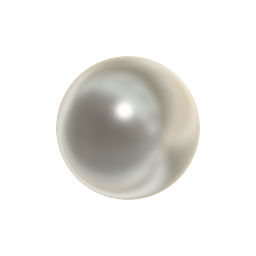
Baby REPO (Autodesk Fusion 360 archive; units mm, degrees)
design "Ojo repo"
Autodesk Fusion 360 part; units mm, degrees
(part 1 of 2)
sphere "EsferaPrimitiva1" add diameter 13 placed x (0, 1, 0) y (0, 0, 1) z (1, 0, 0) at (0, 0, 0)
sketch "Boceto2" plane through (0, 0, 0) normal (0, 1, 0) x (1, 0, 0)
  circle A0 centre (0, 0) radius 20
  dimension "d2" = 40
  constraint coincident A0.centre origin
  measures "d2" diameter of A0
sketch "Boceto1" plane through (0, 0, 0) normal (0, 1, 0) x (1, 0, 0)
  circle A0 centre (0, 0) radius 10
  line L0 (0, 0) -> (0, -13.2142)
  dimension "d1" = 20
  constraint coincident A0.centre L0.start
  constraint vertical L0
  measures "d1" diameter of A0

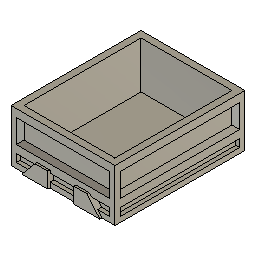
design "Carro"
Autodesk Fusion 360 part; units mm, degrees
sketch "Sketch1" plane through (0, 0, 0) normal (0, 0, 1) x (1, 0, 0)
  line L0 (20, -25) -> (-20, -25)
  line L1 (-20, -25) -> (-20, 25)
  line L2 (-20, 25) -> (20, 25)
  line L3 (20, 25) -> (20, -25)
  line L4 (20, -25) -> (-20, 25) construction
  line L5 (-20, -25) -> (20, 25) construction
  dimension "d1" = 40
  dimension "d2" = 50
  constraint horizontal L0
  constraint perpendicular L0 L1
  constraint parallel L0 L2
  constraint parallel L1 L3
  constraint coincident L4 origin
  constraint coincident L5 origin
  measures "d1" distance of L1.end L2.end
  measures "d2" distance of L0.end L1.end
extrude "Extrude1" add sketch "Sketch1" along normal blind 20
sketch "Sketch2" plane through (0, 25, 0) normal (0, 1, 0) x (-1, 0, 0)
  line L0 (-20, 0) -> (20, 0)
  line L1 (20, 0) -> (20, 20)
  line L2 (20, 20) -> (-20, 20)
  line L3 (-20, 20) -> (-20, 0)
  line L4 (0, 9) -> (0, 20) construction
  line L5 (0, 9) -> (0, 8) construction
  line L6 (0, 8) -> (18, 8)
  line L7 (18, 8) -> (18, 17)
  line L8 (18, 17) -> (-18, 17)
  line L9 (-18, 17) -> (-18, 8)
  line L10 (-18, 8) -> (0, 8)
  line L11 (-18, 8) -> (-18, 2) construction
  line L12 (-18, 2) -> (18, 2) construction
  line L13 (18, 2) -> (18, 8) construction
  line L14 (-18, 2) -> (18, 2)
  line L15 (18, 2) -> (18, 5)
  line L16 (18, 5) -> (-18, 5)
  line L17 (-18, 5) -> (-18, 2)
  line L18 (20, 0) -> (20, 20)
  dimension "d5" = 3
  dimension "d8" = 2
  dimension "d9" = 6
  dimension "d13" = 2
  dimension "d43" = 2
  constraint midpoint L2 L4.end
  constraint perpendicular L0 L4
  constraint coincident L4 L5.end
  constraint perpendicular L5 L6
  constraint perpendicular L6 L7
  constraint perpendicular L4 L8
  constraint perpendicular L6 L9
  constraint perpendicular L5 L10
  constraint perpendicular L10 L11
  constraint perpendicular L11 L12
  constraint perpendicular L12 L13
  constraint horizontal L14
  constraint vertical L15
  constraint horizontal L16
  constraint vertical L17
  constraint midpoint L13 L15.end
  measures "d5" distance of L2 L8
  measures "d8" distance of L3 L9
  measures "d9" distance of L6.end L12.end
  measures "d13" distance of L0 L12
  measures "d43" distance of L7 L18
sketch "Sketch3" plane through (-20, 0, 0) normal (-1, 0, 0) x (0, -1, 0)
  line L0 (-25, 0) -> (25, 0)
  line L1 (25, 0) -> (25, 20)
  line L2 (25, 20) -> (-25, 20)
  line L3 (-25, 20) -> (-25, 0)
  line L4 (-23, 17) -> (23, 17)
  line L5 (23, 17) -> (23, 8)
  line L6 (23, 8) -> (-23, 8)
  line L7 (-23, 8) -> (-23, 17)
  line L8 (-23, 5) -> (23, 5)
  line L9 (23, 5) -> (23, 2)
  line L10 (23, 2) -> (-23, 2)
  line L11 (-23, 2) -> (-23, 5)
  dimension "d14" = 3
  dimension "d15" = 2
  dimension "d16" = 2
  dimension "d18" = 2
  dimension "d19" = 2
  dimension "d20" = 6
  dimension "d21" = 3
  dimension "d22" = 2
  constraint horizontal L4
  constraint vertical L5
  constraint horizontal L6
  constraint vertical L7
  constraint horizontal L8
  constraint vertical L9
  constraint horizontal L10
  constraint vertical L11
  measures "d14" distance of L2 L4
  measures "d15" distance of L1 L5
  measures "d16" distance of L3 L7
  measures "d18" distance of L1 L9
  measures "d19" distance of L3 L11
  measures "d20" distance of L6 L10
  measures "d21" distance of L8 L10
  measures "d22" distance of L0 L10
sketch "Sketch4" plane through (20, 0, 0) normal (1, 0, 0) x (0, 1, 0)
  line L0 (-25, 0) -> (25, 0)
  line L1 (25, 0) -> (25, 20)
  line L2 (25, 20) -> (-25, 20)
  line L3 (-25, 20) -> (-25, 0)
  line L4 (-23, 8) -> (23, 8)
  line L5 (23, 8) -> (23, 17)
  line L6 (-23, 17) -> (-23, 8)
  line L7 (23, 17) -> (-23, 17)
  line L8 (-23, 2) -> (23, 2)
  line L9 (23, 2) -> (23, 5)
  line L10 (-23, 5) -> (-23, 2)
  line L11 (23, 5) -> (-23, 5)
sketch "Sketch5" plane through (0, -25, 0) normal (0, -1, 0) x (1, 0, 0)
  line L0 (-20, 0) -> (20, 0)
  line L1 (20, 0) -> (20, 20)
  line L2 (20, 20) -> (-20, 20)
  line L3 (-20, 20) -> (-20, 0)
  line L4 (-18, 8) -> (-18, 17)
  line L5 (-18, 17) -> (18, 17)
  line L6 (18, 17) -> (18, 8)
  line L7 (0, 8) -> (-18, 8)
  line L8 (18, 8) -> (0, 8)
  line L9 (18, 2) -> (-18, 2)
  line L10 (-18, 2) -> (-18, 5)
  line L11 (18, 5) -> (18, 2)
  line L12 (-18, 5) -> (18, 5)
extrude "Extrude2" cut sketch "Sketch2" against normal blind 1.5 contours L6 L7 L8 L9 L10 | L14 L15 L16 L17
extrude "Extrude3" cut sketch "Sketch3" against normal blind 1.5 contours L4 L5 L6 L7 | L8 L9 L10 L11
extrude "Extrude4" cut sketch "Sketch5" against normal blind 1.5 contours L4 L5 L6 L7 L8 | L9 L10 L11 L12
extrude "Extrude5" cut sketch "Sketch4" against normal blind 1.5 contours L4 L5 L6 L7 | L8 L9 L10 L11
chamfer "Chamfer1" distance 1.5 angle 45 5 edges at (18, 23.5, 12.5) (0, 23.5, 17) (-18, 23.5, 12.5) (0, 23.5, 8) (18.5, 0, 8) 3 faces at (18.5, -7.6667, 14) (-6, -23.5, 14) (-18.5, 7.6667, 14)
sketch "Sketch6" plane through (0, 0, 20) normal (0, 0, 1) x (-1, 0, 0)
  line L0 (-20, -25) -> (20, -25)
  line L1 (20, -25) -> (20, 25)
  line L2 (20, 25) -> (-20, 25)
  line L3 (-20, 25) -> (-20, -25)
  line L4 (-17.5, 22.5) -> (17.5, 22.5)
  line L5 (17.5, 22.5) -> (17.5, -22.5)
  line L6 (17.5, -22.5) -> (-17.5, -22.5)
  line L7 (-17.5, -22.5) -> (-17.5, 22.5)
  line L8 (-17.5, 22.5) -> (17.5, -22.5) construction
  line L9 (17.5, 22.5) -> (-17.5, -22.5) construction
  dimension "d29" = 2.5
  dimension "d30" = 2.5
  constraint horizontal L4
  constraint perpendicular L4 L5
  constraint parallel L4 L6
  constraint parallel L5 L7
  constraint coincident L8 origin
  constraint coincident L9 origin
  measures "d29" distance of L3 L7
  measures "d30" distance of L0 L6
extrude "Extrude6" cut sketch "Sketch6" against normal blind 18 contours L4 L5 L6 L7
sketch "Sketch7" plane through (0, -25, 0) normal (0, -1, 0) x (1, 0, 0)
  line L0 (18, 2) -> (-18, 2)
  line L1 (-18, 5) -> (18, 5)
  line L2 (18, 5) -> (18, 2)
  line L3 (-20, 0) -> (20, 0)
  line L4 (20, 0) -> (20, 20)
  line L5 (20, 20) -> (-20, 20)
  line L6 (-20, 20) -> (-20, 0)
  line L7 (0, 0) -> (0, 20)
  line L8 (0, 0) -> (-5, 0) construction
  line L9 (-5, 0) -> (-5, 6)
  line L10 (-5, 6) -> (-10, 6)
  line L11 (-10, 6) -> (-15, 0)
  line L12 (-5, 0) -> (-15, 0)
  line L13 (10, 6) -> (15, 0)
  line L14 (5, 0) -> (15, 0)
  line L15 (5, 6) -> (10, 6)
  line L16 (5, 0) -> (5, 6)
  line L17 (-18, 17) -> (18, 17)
  line L18 (18, 17) -> (18, 8)
  line L19 (18, 8) -> (-18, 8)
  line L20 (-18, 8) -> (-18, 17)
  line L21 (-18, 2) -> (-18, 5)
  dimension "d33" = 6
  dimension "d34" = 5
  dimension "d35" = 10
  dimension "d36" = 5
  constraint coincident L7.start L8.start
  constraint midpoint L5 L7.end
  constraint coincident L3 L8.end
  constraint perpendicular L1 L9
  constraint perpendicular L9 L10
  constraint coincident L3 L11.end
  constraint symmetric L7 L8.end L14.start
  constraint symmetric L7 L9.end L15.start
  constraint symmetric L7 L10.end L13.start
  constraint symmetric L7 L11.end L13.end
  measures "d33" distance of L8.end L9.end
  measures "d34" distance of L9.end L10.end
  measures "d35" distance of L8.end L11.end
  measures "d36" distance of L7.start L8.end
extrude "Extrude7" add sketch "Sketch7" along normal blind 0.8 and the other way blind 2 contours L0 L3 L13 L14 L16 | L0 L1 L13 L16 | L1 L13 L15 L16 | L0 L3 L9 L11 L12 | L0 L1 L9 L11 | L1 L9 L10 L11
mirror "Mirror1" about plane through (0, 0, 0) normal (0, 1, 0) of "Extrude7"
equation "a = -1.5 mm"
equation "d25 = a"
equation "d27 = a"

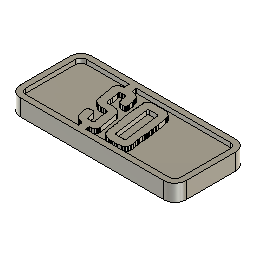
design "Placa"
Autodesk Fusion 360 part; units mm, degrees
sketch "Sketch1" plane through (0, 0, 0) normal (0, 0, 1) x (1, 0, 0)
  line L0 (15, -6.5) -> (-15, -6.5)
  line L1 (-15, -6.5) -> (-15, 6.5)
  line L2 (-15, 6.5) -> (15, 6.5)
  line L3 (15, 6.5) -> (15, -6.5)
  line L4 (15, -6.5) -> (-15, 6.5) construction
  line L5 (-15, -6.5) -> (15, 6.5) construction
  dimension "d1" = 30
  dimension "d2" = 13
  constraint horizontal L0
  constraint perpendicular L0 L1
  constraint parallel L0 L2
  constraint parallel L1 L3
  constraint coincident L4 origin
  constraint coincident L5 origin
  measures "d1" distance of L1.end L2.end
  measures "d2" distance of L0 L2
extrude "Extrude1" add sketch "Sketch1" along normal blind 3
fillet "Fillet1" radius 2 4 edges at (15, 6.5, 1.5) (15, -6.5, 1.5) (-15, 6.5, 1.5) (-15, -6.5, 1.5)
sketch "Sketch2" plane through (0, 0, 3) normal (0, 0, 1) x (-1, 0, 0)
  arc A0 (15, 4.5) -> (13, 6.5) centre (13, 4.5) ccw
  line L0 (13, 6.5) -> (-13, 6.5)
  arc A1 (-13, 6.5) -> (-15, 4.5) centre (-13, 4.5) ccw
  line L1 (-15, 4.5) -> (-15, -4.5)
  arc A2 (-15, -4.5) -> (-13, -6.5) centre (-13, -4.5) ccw
  line L2 (-13, -6.5) -> (13, -6.5)
  arc A3 (13, -6.5) -> (15, -4.5) centre (13, -4.5) ccw
  line L3 (15, -4.5) -> (15, 4.5)
  line L4 (14, -4.5) -> (14, 4.5)
  arc A4 (14, 4.5) -> (13, 5.5) centre (13, 4.5) ccw
  line L5 (13, 5.5) -> (-13, 5.5)
  arc A5 (-13, 5.5) -> (-14, 4.5) centre (-13, 4.5) ccw
  line L6 (-14, 4.5) -> (-14, -4.5)
  arc A6 (-14, -4.5) -> (-13, -5.5) centre (-13, -4.5) ccw
  line L7 (-13, -5.5) -> (13, -5.5)
  arc A7 (13, -5.5) -> (14, -4.5) centre (13, -4.5) ccw
  dimension "d10" = -1
extrude "Extrude2" cut sketch "Sketch2" against normal blind 0.8 contours L4 A4 L5 A5 L6 A6 L7 A7
sketch "Sketch3" plane through (0, 0, 2.2) normal (0, 0, 1) x (-1, 0, 0)
  arc A0 (13, -5.5) -> (14, -4.5) centre (13, -4.5) ccw
  line L0 (14, -4.5) -> (14, 4.5)
  arc A1 (14, 4.5) -> (13, 5.5) centre (13, 4.5) ccw
  line L1 (13, 5.5) -> (-13, 5.5)
  arc A2 (-13, 5.5) -> (-14, 4.5) centre (-13, 4.5) ccw
  line L2 (-14, 4.5) -> (-14, -4.5)
  arc A3 (-14, -4.5) -> (-13, -5.5) centre (-13, -4.5) ccw
  line L3 (-13, -5.5) -> (13, -5.5)
sketch "Sketch5" plane through (0, 0, 2.2) normal (0, 0, 1) x (-1, 0, 0)
  line L0 (-5.6332, -8.2863) -> (-8.0135, 5.2129)
  line L1 (-8.0135, 5.2129) -> (6.4658, 7.766)
  line L2 (6.4658, 7.766) -> (8.8461, -5.7333)
  line L3 (8.8461, -5.7333) -> (-5.6332, -8.2863)
  spline S0 degree 3 poles (3.7042, 3.5054) (3.7183, 3.4541) (3.7488, 3.4163) (3.7582, 3.3648) knots 0 0 0 0 1 1 1 1
  spline S1 degree 2 poles (3.7582, 3.3648) (3.8225, 3.017) (3.9289, 2.3892) knots 0 0 0 1 1 1
  spline S2 degree 2 poles (3.9289, 2.3892) (3.9499, 2.2646) (3.9844, 2.2048) knots 0 0 0 1 1 1
  spline S3 degree 3 poles (3.9844, 2.2048) (4.0535, 2.0848) (4.1345, 2.0478) (4.2734, 1.9569) knots 0 0 0 0 1 1 1 1
  ellipse E0 centre (4.3388, 2.0502) end of major axis (4.228, 2.0165) minor radius 0.1111 (4.2936, 1.9466) -> (4.2734, 1.9569) cw
  spline S4 degree 3 poles (4.2936, 1.9466) (4.3699, 1.917) (4.4549, 1.9046) (4.5418, 1.9217) knots 0 0 0 0 1 1 1 1
  spline S5 degree 3 poles (4.5418, 1.9217) (4.6428, 1.9415) (4.7612, 1.9673) (4.8724, 1.9699) knots 0 0 0 0 1 1 1 1
  ellipse E1 centre (4.8455, 2.1434) end of major axis (4.5703, 2.114) minor radius 0.1754 (4.9108, 1.9765) -> (4.8724, 1.9699) cw
  line L4 (4.9108, 1.9765) -> (5.1509, 2.0309)
  ellipse E2 centre (5.1341, 2.0444) end of major axis (5.1047, 2.0476) minor radius 0.0148 (5.1541, 2.032) -> (5.1509, 2.0309) cw
  spline S6 degree 2 poles (5.1541, 2.032) (5.2823, 2.0818) (5.3138, 2.1979) knots 0 0 0 1 1 1
  spline S7 degree 2 poles (5.3138, 2.1979) (5.3264, 2.2446) (5.3126, 2.3201) knots 0 0 0 1 1 1
  spline S8 degree 2 poles (5.3126, 2.3201) (5.1815, 3.0405) (5.0592, 3.7528) knots 0 0 0 1 1 1
  ellipse E3 centre (4.9332, 3.7277) end of major axis (4.8782, 3.6087) minor radius 0.1271 (5.0447, 3.7941) -> (5.0592, 3.7528) cw
  spline S9 degree 2 poles (5.0447, 3.7941) (5.0017, 3.8706) (4.9904, 3.8877) knots 0 0 0 1 1 1
  spline S10 degree 2 poles (4.9904, 3.8877) (4.9717, 3.9162) (4.8948, 3.9799) knots 0 0 0 1 1 1
  spline S11 degree 2 poles (4.8948, 3.9799) (4.8045, 4.0546) (4.7759, 4.1801) knots 0 0 0 1 1 1
  ellipse E4 centre (4.7092, 4.1685) end of major axis (4.6471, 4.1985) minor radius 0.0652 (4.7695, 4.1969) -> (4.7759, 4.1801) cw
  line L5 (4.7695, 4.1969) -> (4.728, 4.2732)
  ellipse E5 centre (4.6336, 4.2219) end of major axis (4.625, 4.1147) minor radius 0.1074 (4.699, 4.3072) -> (4.728, 4.2732) cw
  spline S12 degree 2 poles (4.699, 4.3072) (4.6777, 4.3217) (4.4902, 4.444) knots 0 0 0 1 1 1
  spline S13 degree 3 poles (4.4902, 4.444) (4.4418, 4.4755) (4.4132, 4.5148) (4.3585, 4.5405) knots 0 0 0 0 1 1 1 1
  spline S14 degree 2 poles (4.3585, 4.5405) (4.2894, 4.5728) (4.2092, 4.6262) knots 0 0 0 1 1 1
  spline S15 degree 3 poles (4.2092, 4.6262) (4.1696, 4.6524) (4.1096, 4.6826) (4.0719, 4.6838) knots 0 0 0 0 1 1 1 1
  spline S16 degree 2 poles (4.0719, 4.6838) (3.9859, 4.6864) (3.9398, 4.6918) knots 0 0 0 1 1 1
  ellipse E6 centre (3.9313, 4.6223) end of major axis (3.8838, 4.5707) minor radius 0.0697 (3.9177, 4.6908) -> (3.9398, 4.6918) cw
  spline S17 degree 3 poles (3.9177, 4.6908) (3.8527, 4.6776) (3.6938, 4.6962) (3.6422, 4.7426) knots 0 0 0 0 1 1 1 1
  spline S18 degree 2 poles (3.6422, 4.7426) (3.6102, 4.7717) (3.5883, 4.8153) knots 0 0 0 1 1 1
  spline S19 degree 2 poles (3.5883, 4.8153) (3.584, 4.8241) (3.548, 4.9034) knots 0 0 0 1 1 1
  ellipse E7 centre (3.6545, 4.9415) end of major axis (3.5521, 5.0009) minor radius 0.1098 (3.548, 4.9034) -> (3.5399, 4.9298) cw
  line L6 (3.5399, 4.9298) -> (3.4522, 5.4189)
  ellipse E8 centre (3.4043, 5.4161) end of major axis (3.3616, 5.4424) minor radius 0.0445 (3.4491, 5.4295) -> (3.4522, 5.4189) cw
  line L7 (3.4491, 5.4295) -> (3.3877, 5.5675)
  ellipse E9 centre (3.3591, 5.5533) end of major axis (3.3543, 5.5206) minor radius 0.0315 (3.3801, 5.5782) -> (3.3877, 5.5675) cw
  spline S20 degree 2 poles (3.3801, 5.5782) (3.2165, 5.7253) (3.1833, 5.7601) knots 0 0 0 1 1 1
  spline S21 degree 3 poles (3.1833, 5.7601) (3.1395, 5.8058) (3.1015, 5.8144) (3.0434, 5.8304) knots 0 0 0 0 1 1 1 1
  spline S22 degree 2 poles (3.0434, 5.8304) (3.0095, 5.8398) (2.9258, 5.8234) knots 0 0 0 1 1 1
  spline S23 degree 2 poles (2.9258, 5.8234) (2.8693, 5.8123) (2.8009, 5.8017) knots 0 0 0 1 1 1
  ellipse E10 centre (2.7856, 5.9348) end of major axis (2.6914, 5.8352) minor radius 0.1319 (2.8009, 5.8017) -> (2.773, 5.8004) cw
  spline S24 degree 2 poles (2.773, 5.8004) (2.6947, 5.8048) (2.6009, 5.7981) knots 0 0 0 1 1 1
  spline S25 degree 2 poles (2.6009, 5.7981) (2.5618, 5.7954) (2.4111, 5.834) knots 0 0 0 1 1 1
  spline S26 degree 3 poles (2.4111, 5.834) (2.374, 5.8436) (2.3396, 5.8315) (2.3143, 5.7961) knots 0 0 0 0 1 1 1 1
  spline S27 degree 2 poles (2.3143, 5.7961) (2.282, 5.7509) (2.2285, 5.7073) knots 0 0 0 1 1 1
  spline S28 degree 2 poles (2.2285, 5.7073) (2.2049, 5.6881) (2.131, 5.584) knots 0 0 0 1 1 1
  ellipse E11 centre (2.1618, 5.5617) end of major axis (2.1476, 5.5972) minor radius 0.0376 (2.1248, 5.5692) -> (2.131, 5.584) cw
  line L8 (2.1248, 5.5692) -> (2.1059, 5.4635)
  ellipse E12 centre (2.122, 5.4609) end of major axis (2.1103, 5.449) minor radius 0.0161 (2.1058, 5.4575) -> (2.1059, 5.4635) cw
  line L9 (2.1058, 5.4575) -> (2.1464, 5.2273)
  ellipse E13 centre (2.2374, 5.2438) end of major axis (2.2002, 5.1588) minor radius 0.0923 (2.1595, 5.1936) -> (2.1464, 5.2273) cw
  spline S29 degree 2 poles (2.1595, 5.1936) (2.1921, 5.1421) (2.1971, 5.1109) knots 0 0 0 1 1 1
  spline S30 degree 3 poles (2.1971, 5.1109) (2.2043, 5.0656) (2.2283, 4.9831) (2.2192, 4.9295) knots 0 0 0 0 1 1 1 1
  spline S31 degree 2 poles (2.2192, 4.9295) (2.2015, 4.826) (2.0854, 4.8045) knots 0 0 0 1 1 1
  spline S32 degree 2 poles (2.0854, 4.8045) (1.8733, 4.7652) (1.7726, 4.75) knots 0 0 0 1 1 1
  spline S33 degree 3 poles (1.7726, 4.75) (1.6587, 4.7331) (1.5681, 4.6825) (1.4836, 4.6125) knots 0 0 0 0 1 1 1 1
  spline S34 degree 3 poles (1.4836, 4.6125) (1.4264, 4.5653) (1.3747, 4.4792) (1.336, 4.4335) knots 0 0 0 0 1 1 1 1
  ellipse E14 centre (1.2733, 4.4643) end of major axis (1.1666, 4.3534) minor radius 0.0673 (1.336, 4.4335) -> (1.3214, 4.4174) cw
  spline S35 degree 2 poles (1.3214, 4.4174) (1.2671, 4.362) (1.2554, 4.3337) knots 0 0 0 1 1 1
  spline S36 degree 2 poles (1.2554, 4.3337) (1.2061, 4.2166) (1.127, 4.1241) knots 0 0 0 1 1 1
  ellipse E15 centre (1.1708, 4.088) end of major axis (1.1151, 4.0731) minor radius 0.0563 (1.1169, 4.107) -> (1.127, 4.1241) cw
  spline S37 degree 2 poles (1.1169, 4.107) (1.0787, 4.0072) (1.0896, 3.9454) knots 0 0 0 1 1 1
  spline S38 degree 2 poles (1.0896, 3.9454) (1.3754, 2.3317) (1.7378, 0.2714) knots 0 0 0 1 1 1
  ellipse E16 centre (1.8383, 0.2915) end of major axis (1.7893, 0.1998) minor radius 0.1016 (1.744, 0.25) -> (1.7378, 0.2714) cw
  spline S39 degree 2 poles (1.744, 0.25) (1.7991, 0.1168) (1.8988, 0.0118) knots 0 0 0 1 1 1
  spline S40 degree 2 poles (1.8988, 0.0118) (1.9758, -0.0691) (2.0755, -0.1635) knots 0 0 0 1 1 1
  ellipse E17 centre (2.116, -0.1214) end of major axis (2.0591, -0.1356) minor radius 0.0578 (2.0972, -0.1763) -> (2.0755, -0.1635) cw
  spline S41 degree 3 poles (2.0972, -0.1763) (2.1797, -0.203) (2.2173, -0.2305) (2.2872, -0.299) knots 0 0 0 0 1 1 1 1
  spline S42 degree 2 poles (2.2872, -0.299) (2.3203, -0.3313) (2.4158, -0.3685) knots 0 0 0 1 1 1
  ellipse E18 centre (2.3546, -0.5014) end of major axis (2.1505, -0.4346) minor radius 0.1457 (2.4158, -0.3685) -> (2.4434, -0.3808) cw
  spline S43 degree 3 poles (2.4434, -0.3808) (2.4902, -0.4046) (2.5404, -0.4499) (2.5956, -0.4682) knots 0 0 0 0 1 1 1 1
  spline S44 degree 2 poles (2.5956, -0.4682) (2.6278, -0.479) (2.6877, -0.4878) knots 0 0 0 1 1 1
  spline S45 degree 2 poles (2.6877, -0.4878) (2.7952, -0.5039) (2.8957, -0.4916) knots 0 0 0 1 1 1
  ellipse E19 centre (2.9106, -0.6007) end of major axis (2.8316, -0.5225) minor radius 0.1085 (2.8957, -0.4916) -> (2.9216, -0.4917) cw
  spline S46 degree 3 poles (2.9216, -0.4917) (3.0151, -0.5031) (3.0801, -0.5057) (3.1705, -0.5306) knots 0 0 0 0 1 1 1 1
  spline S47 degree 3 poles (3.1705, -0.5306) (3.2687, -0.5577) (3.3647, -0.5811) (3.4516, -0.58) knots 0 0 0 0 1 1 1 1
  spline S48 degree 3 poles (3.4516, -0.58) (3.5025, -0.5793) (3.5624, -0.5893) (3.6182, -0.5793) knots 0 0 0 0 1 1 1 1
  spline S49 degree 2 poles (3.6182, -0.5793) (3.7946, -0.5474) (3.9076, -0.5283) knots 0 0 0 1 1 1
  ellipse E20 centre (3.9521, -0.7635) end of major axis (3.7713, -0.604) minor radius 0.2366 (3.9076, -0.5283) -> (3.9622, -0.5253) cw
  spline S50 degree 2 poles (3.9622, -0.5253) (4.059, -0.5312) (4.1472, -0.5134) knots 0 0 0 1 1 1
  ellipse E21 centre (4.1678, -0.6166) end of major axis (4.0909, -0.6891) minor radius 0.1051 (4.1472, -0.5134) -> (4.1947, -0.5147) cw
  spline S51 degree 2 poles (4.1947, -0.5147) (4.3389, -0.5518) (4.4207, -0.6562) knots 0 0 0 1 1 1
  spline S52 degree 2 poles (4.4207, -0.6562) (4.4365, -0.6764) (4.4762, -0.7524) knots 0 0 0 1 1 1
  ellipse E22 centre (4.3194, -0.8307) end of major axis (4.1606, -0.7509) minor radius 0.174 (4.4762, -0.7524) -> (4.4937, -0.8036) cw
  spline S53 degree 2 poles (4.4937, -0.8036) (4.573, -1.2508) (4.6206, -1.5224) knots 0 0 0 1 1 1
  spline S54 degree 3 poles (4.6206, -1.5224) (4.6398, -1.6317) (4.6362, -1.7627) (4.6556, -1.88) knots 0 0 0 0 1 1 1 1
  spline S55 degree 2 poles (4.6556, -1.88) (4.7234, -2.2878) (4.8534, -2.9942) knots 0 0 0 1 1 1
  spline S56 degree 2 poles (4.8534, -2.9942) (4.86, -3.0309) (4.8753, -3.1323) knots 0 0 0 1 1 1
  spline S57 degree 2 poles (4.8753, -3.1323) (4.8871, -3.2112) (4.8746, -3.2397) knots 0 0 0 1 1 1
  spline S58 degree 2 poles (4.8746, -3.2397) (4.8522, -3.2907) (4.7914, -3.3065) knots 0 0 0 1 1 1
  spline S59 degree 2 poles (4.7914, -3.3065) (4.6593, -3.3404) (4.5362, -3.3464) knots 0 0 0 1 1 1
  spline S60 degree 2 poles (4.5362, -3.3464) (4.3964, -3.3533) (4.3296, -3.3641) knots 0 0 0 1 1 1
  spline S61 degree 2 poles (4.3296, -3.3641) (4.2017, -3.3849) (4.1214, -3.3989) knots 0 0 0 1 1 1
  ellipse E23 centre (4.1007, -3.2842) end of major axis (4.0144, -3.2057) minor radius 0.1162 (4.1214, -3.3989) -> (4.0915, -3.4003) cw
  spline S62 degree 2 poles (4.0915, -3.4003) (4.0313, -3.3957) (3.9947, -3.3961) knots 0 0 0 1 1 1
  spline S63 degree 3 poles (3.9947, -3.3961) (3.8881, -3.397) (3.7772, -3.336) (3.7223, -3.2494) knots 0 0 0 0 1 1 1 1
  spline S64 degree 3 poles (3.7223, -3.2494) (3.6918, -3.2016) (3.6734, -3.1397) (3.6476, -3.0836) knots 0 0 0 0 1 1 1 1
  ellipse E24 centre (3.8265, -3.0007) end of major axis (3.7362, -3.1763) minor radius 0.1968 (3.6476, -3.0836) -> (3.633, -3.0381) cw
  spline S65 degree 2 poles (3.633, -3.0381) (3.551, -2.5949) (3.4919, -2.236) knots 0 0 0 1 1 1
  spline S66 degree 2 poles (3.4919, -2.236) (3.4829, -2.181) (3.4574, -2.1283) knots 0 0 0 1 1 1
  spline S67 degree 3 poles (3.4574, -2.1283) (3.4329, -2.0772) (3.4312, -2.055) (3.4185, -1.9978) knots 0 0 0 0 1 1 1 1
  ellipse E25 centre (3.3433, -2.0132) end of major axis (3.2734, -1.9805) minor radius 0.0758 (3.4111, -1.9781) -> (3.4185, -1.9978) cw
  spline S68 degree 2 poles (3.4111, -1.9781) (3.3725, -1.9071) (3.3356, -1.8544) knots 0 0 0 1 1 1
  spline S69 degree 3 poles (3.3356, -1.8544) (3.2537, -1.7372) (3.1819, -1.6361) (3.0209, -1.6632) knots 0 0 0 0 1 1 1 1
  spline S70 degree 3 poles (3.0209, -1.6632) (2.9052, -1.6828) (2.7507, -1.6363) (2.6492, -1.592) knots 0 0 0 0 1 1 1 1
  spline S71 degree 2 poles (2.6492, -1.592) (2.6322, -1.5846) (2.5234, -1.5736) knots 0 0 0 1 1 1
  spline S72 degree 3 poles (2.5234, -1.5736) (2.4418, -1.5651) (2.371, -1.5894) (2.284, -1.6019) knots 0 0 0 0 1 1 1 1
  spline S73 degree 2 poles (2.284, -1.6019) (2.223, -1.6107) (2.1768, -1.6373) knots 0 0 0 1 1 1
  spline S74 degree 2 poles (2.1768, -1.6373) (2.1141, -1.6735) (2.0939, -1.7329) knots 0 0 0 1 1 1
  spline S75 degree 2 poles (2.0939, -1.7329) (2.0484, -1.8673) (2.034, -2.0334) knots 0 0 0 1 1 1
  ellipse E26 centre (2.2426, -2.0524) end of major axis (2.0881, -1.9104) minor radius 0.2088 (2.0364, -2.0878) -> (2.034, -2.0334) cw
  line L10 (2.0364, -2.0878) -> (2.0588, -2.2147)
  ellipse E27 centre (2.0103, -2.2292) end of major axis (1.9774, -2.2705) minor radius 0.0469 (2.0588, -2.2147) -> (2.0594, -2.2267) cw
  spline S76 degree 2 poles (2.0594, -2.2267) (2.0551, -2.3184) (2.0613, -2.3619) knots 0 0 0 1 1 1
  spline S77 degree 2 poles (2.0613, -2.3619) (2.098, -2.621) (2.1839, -3.0777) knots 0 0 0 1 1 1
  spline S78 degree 2 poles (2.1839, -3.0777) (2.1874, -3.0968) (2.2096, -3.1391) knots 0 0 0 1 1 1
  ellipse E28 centre (1.986, -3.2542) end of major axis (1.7602, -3.1416) minor radius 0.2509 (2.2096, -3.1391) -> (2.2344, -3.2128) cw
  spline S79 degree 3 poles (2.2344, -3.2128) (2.2407, -3.2481) (2.2462, -3.2843) (2.2631, -3.3219) knots 0 0 0 0 1 1 1 1
  spline S80 degree 2 poles (2.2631, -3.3219) (2.3377, -3.4886) (2.3795, -3.5706) knots 0 0 0 1 1 1
  ellipse E29 centre (2.2738, -3.6299) end of major axis (2.2198, -3.74) minor radius 0.1185 (2.3795, -3.5706) -> (2.3917, -3.608) cw
  spline S81 degree 2 poles (2.3917, -3.608) (2.4032, -3.6818) (2.4392, -3.7447) knots 0 0 0 1 1 1
  ellipse E30 centre (2.35, -3.7926) end of major axis (2.2574, -3.7488) minor radius 0.1006 (2.4392, -3.7447) -> (2.4502, -3.7746) cw
  line L11 (2.4502, -3.7746) -> (2.4688, -3.8728)
  ellipse E31 centre (2.4923, -3.869) end of major axis (2.4709, -3.8583) minor radius 0.0236 (2.4712, -3.8797) -> (2.4688, -3.8728) cw
  spline S82 degree 2 poles (2.4712, -3.8797) (2.5203, -3.979) (2.5632, -4.0262) knots 0 0 0 1 1 1
  spline S83 degree 2 poles (2.5632, -4.0262) (2.6772, -4.1515) (2.7849, -4.2633) knots 0 0 0 1 1 1
  spline S84 degree 2 poles (2.7849, -4.2633) (2.8153, -4.2948) (2.9061, -4.3287) knots 0 0 0 1 1 1
  ellipse E32 centre (2.8607, -4.4056) end of major axis (2.7566, -4.4082) minor radius 0.0851 (2.9061, -4.3287) -> (2.9189, -4.3346) cw
  spline S85 degree 2 poles (2.9189, -4.3346) (3.1219, -4.4422) (3.1701, -4.4557) knots 0 0 0 1 1 1
  spline S86 degree 2 poles (3.1701, -4.4557) (3.2025, -4.4648) (3.3011, -4.4853) knots 0 0 0 1 1 1
  spline S87 degree 2 poles (3.3011, -4.4853) (3.4081, -4.5076) (3.5643, -4.5661) knots 0 0 0 1 1 1
  spline S88 degree 2 poles (3.5643, -4.5661) (3.6374, -4.5935) (3.7703, -4.6108) knots 0 0 0 1 1 1
  ellipse E33 centre (3.7616, -4.6673) end of major axis (3.7083, -4.6908) minor radius 0.0567 (3.7703, -4.6108) -> (3.7947, -4.6199) cw
  spline S89 degree 2 poles (3.7947, -4.6199) (3.8598, -4.6619) (3.8726, -4.7279) knots 0 0 0 1 1 1
  spline S90 degree 2 poles (3.8726, -4.7279) (3.903, -4.8834) (3.9865, -5.37) knots 0 0 0 1 1 1
  ellipse E34 centre (4.0733, -5.3621) end of major axis (3.9959, -5.3174) minor radius 0.0831 (3.9934, -5.3924) -> (3.9865, -5.37) cw
  spline S91 degree 2 poles (3.9934, -5.3924) (4.0073, -5.4235) (4.048, -5.5018) knots 0 0 0 1 1 1
  spline S92 degree 2 poles (4.048, -5.5018) (4.0709, -5.5457) (4.1079, -5.5696) knots 0 0 0 1 1 1
  spline S93 degree 2 poles (4.1079, -5.5696) (4.2419, -5.6567) (4.3152, -5.7037) knots 0 0 0 1 1 1
  spline S94 degree 3 poles (4.3152, -5.7037) (4.3836, -5.7476) (4.4312, -5.732) (4.4945, -5.7443) knots 0 0 0 0 1 1 1 1
  ellipse E35 centre (4.5109, -5.6478) end of major axis (4.4413, -5.576) minor radius 0.0968 (4.5273, -5.7454) -> (4.4945, -5.7443) cw
  line L12 (4.5273, -5.7454) -> (4.6225, -5.7323)
  ellipse E36 centre (4.6259, -5.7533) end of major axis (4.6108, -5.7379) minor radius 0.0207 (4.6225, -5.7323) -> (4.6289, -5.7325) cw
  spline S95 degree 2 poles (4.6289, -5.7325) (4.6896, -5.7459) (4.7868, -5.7288) knots 0 0 0 1 1 1
  spline S96 degree 2 poles (4.7868, -5.7288) (5.0441, -5.6831) (5.0633, -5.6795) knots 0 0 0 1 1 1
  spline S97 degree 3 poles (5.0633, -5.6795) (5.1606, -5.6611) (5.2388, -5.5537) (5.2685, -5.4662) knots 0 0 0 0 1 1 1 1
  spline S98 degree 2 poles (5.2685, -5.4662) (5.2767, -5.4424) (5.2868, -5.3368) knots 0 0 0 1 1 1
  ellipse E37 centre (5.1554, -5.3198) end of major axis (5.0582, -5.227) minor radius 0.1294 (5.2853, -5.3017) -> (5.2868, -5.3368) cw
  spline S99 degree 2 poles (5.2853, -5.3017) (5.2348, -5.0176) (5.1897, -4.7651) knots 0 0 0 1 1 1
  spline S100 degree 2 poles (5.1897, -4.7651) (5.1856, -4.7418) (5.2069, -4.637) knots 0 0 0 1 1 1
  ellipse E38 centre (5.2466, -4.6455) end of major axis (5.2338, -4.6068) minor radius 0.0404 (5.2069, -4.637) -> (5.2163, -4.6182) cw
  spline S101 degree 2 poles (5.2163, -4.6182) (5.2679, -4.5606) (5.3091, -4.551) knots 0 0 0 1 1 1
  spline S102 degree 3 poles (5.3091, -4.551) (5.349, -4.5417) (5.4116, -4.533) (5.4627, -4.508) knots 0 0 0 0 1 1 1 1
  spline S103 degree 2 poles (5.4627, -4.508) (5.5138, -4.4832) (5.5295, -4.4817) knots 0 0 0 1 1 1
  spline S104 degree 2 poles (5.5295, -4.4817) (5.6497, -4.4701) (5.7409, -4.4244) knots 0 0 0 1 1 1
  ellipse E39 centre (5.7899, -4.5277) end of major axis (5.7392, -4.6316) minor radius 0.1136 (5.7409, -4.4244) -> (5.7665, -4.4153) cw
  spline S105 degree 2 poles (5.7665, -4.4153) (5.8986, -4.3853) (5.9949, -4.2875) knots 0 0 0 1 1 1
  spline S106 degree 2 poles (5.9949, -4.2875) (6.0482, -4.2335) (6.0813, -4.2025) knots 0 0 0 1 1 1
  spline S107 degree 3 poles (6.0813, -4.2025) (6.1992, -4.0926) (6.2796, -3.9513) (6.3271, -3.7951) knots 0 0 0 0 1 1 1 1
  spline S108 degree 3 poles (6.3271, -3.7951) (6.3466, -3.7313) (6.3424, -3.6802) (6.3519, -3.6138) knots 0 0 0 0 1 1 1 1
  ellipse E40 centre (6.2447, -3.6027) end of major axis (6.1693, -3.6835) minor radius 0.1064 (6.3513, -3.58) -> (6.3519, -3.6138) cw
  line L13 (6.3513, -3.58) -> (5.8761, -0.8846)
  ellipse E41 centre (5.9518, -0.8674) end of major axis (5.9004, -0.9276) minor radius 0.0753 (5.8761, -0.8846) -> (5.8751, -0.8661) cw
  spline S109 degree 3 poles (5.8751, -0.8661) (5.8845, -0.7303) (5.8483, -0.5717) (5.8087, -0.4493) knots 0 0 0 0 1 1 1 1
  spline S110 degree 3 poles (5.8087, -0.4493) (5.7818, -0.3658) (5.7747, -0.2939) (5.7571, -0.2119) knots 0 0 0 0 1 1 1 1
  ellipse E42 centre (5.7028, -0.2257) end of major axis (5.6805, -0.2786) minor radius 0.0552 (5.7508, -0.1954) -> (5.7571, -0.2119) cw
  spline S111 degree 2 poles (5.7508, -0.1954) (5.6709, -0.0529) (5.6494, -0.0316) knots 0 0 0 1 1 1
  spline S112 degree 2 poles (5.6494, -0.0316) (5.5725, 0.045) (5.4718, 0.1591) knots 0 0 0 1 1 1
  spline S113 degree 2 poles (5.4718, 0.1591) (5.4545, 0.1788) (5.3635, 0.2335) knots 0 0 0 1 1 1
  spline S114 degree 2 poles (5.3635, 0.2335) (5.3037, 0.2696) (5.2591, 0.3008) knots 0 0 0 1 1 1
  spline S115 degree 2 poles (5.2591, 0.3008) (5.1959, 0.345) (4.9601, 0.4972) knots 0 0 0 1 1 1
  spline S116 degree 3 poles (4.9601, 0.4972) (4.9043, 0.5333) (4.8381, 0.557) (4.7799, 0.5642) knots 0 0 0 0 1 1 1 1
  spline S117 degree 3 poles (4.7799, 0.5642) (4.6185, 0.5839) (4.4655, 0.6427) (4.3178, 0.6727) knots 0 0 0 0 1 1 1 1
  spline S118 degree 2 poles (4.3178, 0.6727) (4.2982, 0.6768) (4.1971, 0.6702) knots 0 0 0 1 1 1
  ellipse E43 centre (4.1832, 0.761) end of major axis (4.1147, 0.8276) minor radius 0.0865 (4.1971, 0.6702) -> (4.1809, 0.6708) cw
  spline S119 degree 2 poles (4.1809, 0.6708) (4.1197, 0.6784) (4.0582, 0.6679) knots 0 0 0 1 1 1
  spline S120 degree 2 poles (4.0582, 0.6679) (3.9525, 0.6497) (3.8299, 0.6287) knots 0 0 0 1 1 1
  ellipse E44 centre (3.8207, 0.6594) end of major axis (3.7946, 0.6802) minor radius 0.0295 (3.8299, 0.6287) -> (3.8221, 0.6284) cw
  line L14 (3.8221, 0.6284) -> (3.7471, 0.6327)
  ellipse E45 centre (3.739, 0.4879) end of major axis (3.6399, 0.3816) minor radius 0.1448 (3.7215, 0.6318) -> (3.7471, 0.6327) cw
  spline S121 degree 2 poles (3.7215, 0.6318) (3.6025, 0.6162) (3.5175, 0.6323) knots 0 0 0 1 1 1
  spline S122 degree 2 poles (3.5175, 0.6323) (3.3331, 0.6676) (3.2055, 0.6771) knots 0 0 0 1 1 1
  spline S123 degree 3 poles (3.2055, 0.6771) (3.1141, 0.6839) (3.066, 0.7027) (3.0125, 0.7666) knots 0 0 0 0 1 1 1 1
  spline S124 degree 2 poles (3.0125, 0.7666) (2.9822, 0.8028) (2.9649, 0.9055) knots 0 0 0 1 1 1
  spline S125 degree 2 poles (2.9649, 0.9055) (2.92, 1.1739) (2.9067, 1.2519) knots 0 0 0 1 1 1
  ellipse E46 centre (3.0716, 1.2827) end of major axis (2.9589, 1.1576) minor radius 0.1666 (2.9067, 1.2519) -> (2.9047, 1.2946) cw
  spline S126 degree 2 poles (2.9047, 1.2946) (2.9114, 1.3769) (2.8908, 1.4922) knots 0 0 0 1 1 1
  spline S127 degree 2 poles (2.8908, 1.4922) (2.7057, 2.5294) (2.5642, 3.3458) knots 0 0 0 1 1 1
  ellipse E47 centre (2.7505, 3.3837) end of major axis (2.6222, 3.2403) minor radius 0.186 (2.5642, 3.3458) -> (2.5624, 3.3944) cw
  spline S128 degree 3 poles (2.5624, 3.3944) (2.5714, 3.4975) (2.5616, 3.6208) (2.6941, 3.6417) knots 0 0 0 0 1 1 1 1
  spline S129 degree 2 poles (2.6941, 3.6417) (2.7331, 3.6478) (2.8708, 3.6647) knots 0 0 0 1 1 1
  ellipse E48 centre (2.888, 3.5091) end of major axis (2.7763, 3.3989) minor radius 0.1563 (2.8708, 3.6647) -> (2.9078, 3.6646) cw
  line L15 (2.9078, 3.6646) -> (2.952, 3.659)
  ellipse E49 centre (2.9573, 3.7268) end of major axis (2.905, 3.7735) minor radius 0.0668 (2.9734, 3.6597) -> (2.952, 3.659) cw
  spline S130 degree 2 poles (2.9734, 3.6597) (3.028, 3.6696) (3.0775, 3.6644) knots 0 0 0 1 1 1
  spline S131 degree 3 poles (3.0775, 3.6644) (3.1571, 3.6557) (3.2316, 3.676) (3.3093, 3.6902) knots 0 0 0 0 1 1 1 1
  spline S132 degree 3 poles (3.3093, 3.6902) (3.3534, 3.6983) (3.4033, 3.6838) (3.4511, 3.6883) knots 0 0 0 0 1 1 1 1
  spline S133 degree 3 poles (3.4511, 3.6883) (3.5036, 3.6932) (3.5798, 3.6804) (3.6163, 3.6396) knots 0 0 0 0 1 1 1 1
  spline S134 degree 2 poles (3.6163, 3.6396) (3.669, 3.5806) (3.6984, 3.5206) knots 0 0 0 1 1 1
  ellipse E50 centre (3.6258, 3.4721) end of major axis (3.5938, 3.386) minor radius 0.0804 (3.6984, 3.5206) -> (3.7042, 3.5054) cw
  line L16 (-0.2429, -4.6585) -> (-0.1268, -4.6633)
  ellipse E51 centre (-0.1233, -4.6145) end of major axis (-0.1565, -4.6513) minor radius 0.048 (-0.1164, -4.6626) -> (-0.1268, -4.6633) cw
  line L17 (-0.1164, -4.6626) -> (0.178, -4.6107)
  ellipse E52 centre (0.1745, -4.5712) end of major axis (0.1525, -4.6059) minor radius 0.0376 (0.1848, -4.6089) -> (0.178, -4.6107) cw
  line L18 (0.1848, -4.6089) -> (0.3598, -4.5446)
  ellipse E53 centre (0.3425, -4.5175) end of major axis (0.3079, -4.5089) minor radius 0.0292 (0.3641, -4.5425) -> (0.3598, -4.5446) cw
  spline S135 degree 3 poles (0.3641, -4.5425) (0.3995, -4.5216) (0.4254, -4.5083) (0.4522, -4.4867) knots 0 0 0 0 1 1 1 1
  spline S136 degree 2 poles (0.4522, -4.4867) (0.5599, -4.4003) (0.7494, -4.2762) knots 0 0 0 1 1 1
  spline S137 degree 2 poles (0.7494, -4.2762) (0.7796, -4.2564) (0.8197, -4.2074) knots 0 0 0 1 1 1
  spline S138 degree 3 poles (0.8197, -4.2074) (0.9121, -4.0945) (0.9814, -3.977) (1.0208, -3.8413) knots 0 0 0 0 1 1 1 1
  spline S139 degree 2 poles (1.0208, -3.8413) (1.03, -3.8093) (1.0174, -3.7503) knots 0 0 0 1 1 1
  spline S140 degree 2 poles (1.0174, -3.7503) (1.0003, -3.6721) (1.0042, -3.5823) knots 0 0 0 1 1 1
  ellipse E54 centre (0.9262, -3.5797) end of major axis (0.8743, -3.6384) minor radius 0.0778 (1.0033, -3.5673) -> (1.0042, -3.5823) cw
  line L19 (1.0033, -3.5673) -> (0.8623, -2.6881)
  ellipse E55 centre (0.8919, -2.6805) end of major axis (0.8707, -2.7036) minor radius 0.0289 (0.8623, -2.6881) -> (0.8623, -2.6778) cw
  spline S141 degree 2 poles (0.8623, -2.6778) (0.874, -2.6089) (0.8651, -2.5605) knots 0 0 0 1 1 1
  spline S142 degree 3 poles (0.8651, -2.5605) (0.8568, -2.5145) (0.874, -2.4657) (0.8691, -2.4243) knots 0 0 0 0 1 1 1 1
  spline S143 degree 2 poles (0.8691, -2.4243) (0.8646, -2.386) (0.8713, -2.3224) knots 0 0 0 1 1 1
  spline S144 degree 2 poles (0.8713, -2.3224) (0.8755, -2.2838) (0.8639, -2.2083) knots 0 0 0 1 1 1
  ellipse E56 centre (0.9233, -2.2) end of major axis (0.8798, -2.158) minor radius 0.0595 (0.8639, -2.2083) -> (0.8635, -2.193) cw
  line L20 (0.8635, -2.193) -> (0.8716, -2.1105)
  ellipse E57 centre (0.8645, -2.1085) end of major axis (0.859, -2.103) minor radius 0.0067 (0.8714, -2.1074) -> (0.8716, -2.1105) cw
  spline S145 degree 2 poles (0.8714, -2.1074) (0.8584, -2.0445) (0.8635, -1.9957) knots 0 0 0 1 1 1
  spline S146 degree 3 poles (0.8635, -1.9957) (0.8724, -1.9123) (0.8579, -1.8552) (0.8429, -1.7689) knots 0 0 0 0 1 1 1 1
  ellipse E58 centre (1.0207, -1.7339) end of major axis (0.899, -1.87) minor radius 0.179 (0.8429, -1.7689) -> (0.8407, -1.7226) cw
  spline S147 degree 2 poles (0.8407, -1.7226) (0.8484, -1.6337) (0.8381, -1.5795) knots 0 0 0 1 1 1
  spline S148 degree 2 poles (0.8381, -1.5795) (0.8276, -1.5233) (0.7594, -1.1282) knots 0 0 0 1 1 1
  ellipse E59 centre (0.9686, -1.0926) end of major axis (0.8105, -0.9498) minor radius 0.2117 (0.7594, -1.1282) -> (0.7567, -1.0767) cw
  spline S149 degree 2 poles (0.7567, -1.0767) (0.7629, -0.9856) (0.7454, -0.8864) knots 0 0 0 1 1 1
  spline S150 degree 2 poles (0.7454, -0.8864) (0.3063, 1.6024) (0.2939, 1.676) knots 0 0 0 1 1 1
  ellipse E60 centre (0.5232, 1.7345) end of major axis (0.3744, 1.54) minor radius 0.2249 (0.2939, 1.676) -> (0.2908, 1.7116) cw
  spline S151 degree 2 poles (0.2908, 1.7116) (0.2898, 1.8399) (0.2831, 1.8718) knots 0 0 0 1 1 1
  spline S152 degree 2 poles (0.2831, 1.8718) (0.2389, 2.079) (0.162, 2.4861) knots 0 0 0 1 1 1
  spline S153 degree 2 poles (0.162, 2.4861) (0.1513, 2.5431) (0.142, 2.6151) knots 0 0 0 1 1 1
  spline S154 degree 2 poles (0.142, 2.6151) (0.1364, 2.6583) (0.1246, 2.7444) knots 0 0 0 1 1 1
  spline S155 degree 2 poles (0.1246, 2.7444) (0.0818, 3.0612) (-0.0439, 3.7455) knots 0 0 0 1 1 1
  spline S156 degree 2 poles (-0.0439, 3.7455) (-0.0481, 3.7681) (-0.0742, 3.8277) knots 0 0 0 1 1 1
  spline S157 degree 3 poles (-0.0742, 3.8277) (-0.1065, 3.9016) (-0.1074, 3.9501) (-0.1273, 4.0596) knots 0 0 0 0 1 1 1 1
  ellipse E61 centre (-0.2332, 4.0352) end of major axis (-0.2818, 3.935) minor radius 0.1069 (-0.1359, 4.0861) -> (-0.1273, 4.0596) cw
  spline S158 degree 3 poles (-0.1359, 4.0861) (-0.18, 4.1782) (-0.2372, 4.2744) (-0.3262, 4.3521) knots 0 0 0 0 1 1 1 1
  spline S159 degree 2 poles (-0.3262, 4.3521) (-0.3611, 4.3824) (-0.4548, 4.4769) knots 0 0 0 1 1 1
  ellipse E62 centre (-0.5415, 4.3921) end of major axis (-0.6621, 4.3773) minor radius 0.1209 (-0.4796, 4.4962) -> (-0.4548, 4.4769) cw
  spline S160 degree 2 poles (-0.4796, 4.4962) (-0.6213, 4.5807) (-0.7023, 4.6548) knots 0 0 0 1 1 1
  ellipse E63 centre (-0.8094, 4.5359) end of major axis (-0.8431, 4.6931) minor radius 0.1595 (-0.7458, 4.6831) -> (-0.7023, 4.6548) cw
  spline S161 degree 2 poles (-0.7458, 4.6831) (-0.843, 4.726) (-0.9509, 4.8047) knots 0 0 0 1 1 1
  spline S162 degree 3 poles (-0.9509, 4.8047) (-1.0484, 4.8759) (-1.1751, 4.884) (-1.2879, 4.906) knots 0 0 0 0 1 1 1 1
  ellipse E64 centre (-1.2277, 5.2287) end of major axis (-1.3866, 5.5178) minor radius 0.326 (-1.2879, 4.906) -> (-1.3455, 4.9231) cw
  spline S163 degree 3 poles (-1.3455, 4.9231) (-1.4546, 4.9671) (-1.6108, 5.0143) (-1.7181, 5.0027) knots 0 0 0 0 1 1 1 1
  spline S164 degree 2 poles (-1.7181, 5.0027) (-1.7706, 4.9971) (-1.8543, 4.9802) knots 0 0 0 1 1 1
  spline S165 degree 2 poles (-1.8543, 4.9802) (-1.8782, 4.9753) (-1.9619, 4.9759) knots 0 0 0 1 1 1
  spline S166 degree 3 poles (-1.9619, 4.9759) (-2.0499, 4.9764) (-2.17, 4.9524) (-2.2256, 4.9415) knots 0 0 0 0 1 1 1 1
  spline S167 degree 3 poles (-2.2256, 4.9415) (-2.3063, 4.9258) (-2.4169, 4.9327) (-2.4735, 4.9589) knots 0 0 0 0 1 1 1 1
  spline S168 degree 3 poles (-2.4735, 4.9589) (-2.598, 5.0164) (-2.7075, 5.025) (-2.843, 4.9972) knots 0 0 0 0 1 1 1 1
  spline S169 degree 2 poles (-2.843, 4.9972) (-2.8781, 4.99) (-2.987, 4.9902) knots 0 0 0 1 1 1
  spline S170 degree 2 poles (-2.987, 4.9902) (-3.0182, 4.9903) (-3.0474, 4.9859) knots 0 0 0 1 1 1
  spline S171 degree 2 poles (-3.0474, 4.9859) (-3.1024, 4.9779) (-3.7272, 4.8664) knots 0 0 0 1 1 1
  spline S172 degree 2 poles (-3.7272, 4.8664) (-3.758, 4.861) (-3.8436, 4.826) knots 0 0 0 1 1 1
  ellipse E65 centre (-3.9074, 4.9646) end of major axis (-4.0453, 5.0348) minor radius 0.1493 (-3.8436, 4.826) -> (-3.8728, 4.8171) cw
  spline S173 degree 3 poles (-3.8728, 4.8171) (-3.9744, 4.7964) (-4.0535, 4.7929) (-4.1401, 4.7137) knots 0 0 0 0 1 1 1 1
  ellipse E66 centre (-4.0936, 4.6607) end of major axis (-4.1066, 4.7305) minor radius 0.0695 (-4.1587, 4.686) -> (-4.1401, 4.7137) cw
  spline S174 degree 3 poles (-4.1587, 4.686) (-4.1691, 4.6578) (-4.1835, 4.6249) (-4.2053, 4.5961) knots 0 0 0 0 1 1 1 1
  spline S175 degree 2 poles (-4.2053, 4.5961) (-4.248, 4.54) (-4.2995, 4.4723) knots 0 0 0 1 1 1
  ellipse E67 centre (-4.1555, 4.3628) end of major axis (-4.329, 4.311) minor radius 0.1809 (-4.3262, 4.4229) -> (-4.2995, 4.4723) cw
  line L21 (-4.3262, 4.4229) -> (-4.373, 4.29)
  ellipse E68 centre (-4.4432, 4.3186) end of major axis (-4.4661, 4.3932) minor radius 0.0745 (-4.373, 4.29) -> (-4.3813, 4.2734) cw
  spline S176 degree 3 poles (-4.3813, 4.2734) (-4.4268, 4.2036) (-4.4664, 4.1237) (-4.465, 4.0417) knots 0 0 0 0 1 1 1 1
  spline S177 degree 3 poles (-4.465, 4.0417) (-4.4634, 3.9479) (-4.4738, 3.9099) (-4.4575, 3.8189) knots 0 0 0 0 1 1 1 1
  spline S178 degree 3 poles (-4.4575, 3.8189) (-4.4391, 3.7167) (-4.3939, 3.5036) (-4.3876, 3.3414) knots 0 0 0 0 1 1 1 1
  spline S179 degree 2 poles (-4.3876, 3.3414) (-4.3814, 3.1835) (-4.3338, 3.036) knots 0 0 0 1 1 1
  spline S180 degree 2 poles (-4.3338, 3.036) (-4.2999, 2.9317) (-4.2892, 2.8676) knots 0 0 0 1 1 1
  spline S181 degree 2 poles (-4.2892, 2.8676) (-4.263, 2.7098) (-4.2343, 2.5544) knots 0 0 0 1 1 1
  spline S182 degree 2 poles (-4.2343, 2.5544) (-4.2213, 2.484) (-4.214, 2.3485) knots 0 0 0 1 1 1
  spline S183 degree 2 poles (-4.214, 2.3485) (-4.2073, 2.2219) (-4.1791, 2.0833) knots 0 0 0 1 1 1
  spline S184 degree 2 poles (-4.1791, 2.0833) (-4.166, 2.0193) (-4.0672, 1.4411) knots 0 0 0 1 1 1
  ellipse E69 centre (-4.2448, 1.4073) end of major axis (-4.3682, 1.274) minor radius 0.1791 (-4.0672, 1.4411) -> (-4.0656, 1.3896) cw
  spline S185 degree 2 poles (-4.0656, 1.3896) (-4.0768, 1.2887) (-4.0895, 1.113) knots 0 0 0 1 1 1
  spline S186 degree 3 poles (-4.0895, 1.113) (-4.0916, 1.0841) (-4.0882, 1.0686) (-4.0838, 1.0306) knots 0 0 0 0 1 1 1 1
  ellipse E70 centre (-4.2689, 1.008) end of major axis (-4.4025, 0.8772) minor radius 0.1857 (-4.0838, 1.0306) -> (-4.0845, 0.9827) cw
  spline S187 degree 3 poles (-4.0845, 0.9827) (-4.0943, 0.9125) (-4.0835, 0.868) (-4.069, 0.7768) knots 0 0 0 0 1 1 1 1
  ellipse E71 centre (-4.14, 0.7649) end of major axis (-4.1915, 0.7145) minor radius 0.0717 (-4.069, 0.7768) -> (-4.0694, 0.7518) cw
  spline S188 degree 2 poles (-4.0694, 0.7518) (-4.0811, 0.6881) (-4.0608, 0.5783) knots 0 0 0 1 1 1
  spline S189 degree 2 poles (-4.0608, 0.5783) (-4.0582, 0.5644) (-4.0162, 0.3192) knots 0 0 0 1 1 1
  spline S190 degree 2 poles (-4.0162, 0.3192) (-4.0119, 0.2939) (-4.0146, 0.2342) knots 0 0 0 1 1 1
  spline S191 degree 3 poles (-4.0146, 0.2342) (-4.0169, 0.1862) (-4.0108, 0.1386) (-4.0047, 0.1012) knots 0 0 0 0 1 1 1 1
  spline S192 degree 2 poles (-4.0047, 0.1012) (-3.9862, -0.0128) (-3.9186, -0.3923) knots 0 0 0 1 1 1
  spline S193 degree 2 poles (-3.9186, -0.3923) (-3.905, -0.4688) (-3.9048, -0.553) knots 0 0 0 1 1 1
  spline S194 degree 2 poles (-3.9048, -0.553) (-3.9044, -0.6385) (-3.8784, -0.7852) knots 0 0 0 1 1 1
  spline S195 degree 2 poles (-3.8784, -0.7852) (-3.8704, -0.8294) (-3.8189, -1.1194) knots 0 0 0 1 1 1
  spline S196 degree 2 poles (-3.8189, -1.1194) (-3.7984, -1.2348) (-3.7802, -1.4169) knots 0 0 0 1 1 1
  spline S197 degree 2 poles (-3.7802, -1.4169) (-3.7643, -1.5766) (-3.7414, -1.7147) knots 0 0 0 1 1 1
  spline S198 degree 2 poles (-3.7414, -1.7147) (-3.6783, -2.0981) (-3.4693, -3.2411) knots 0 0 0 1 1 1
  spline S199 degree 3 poles (-3.4693, -3.2411) (-3.456, -3.3139) (-3.4163, -3.4049) (-3.4027, -3.4828) knots 0 0 0 0 1 1 1 1
  spline S200 degree 2 poles (-3.4027, -3.4828) (-3.3844, -3.5875) (-3.3465, -3.8069) knots 0 0 0 1 1 1
  ellipse E72 centre (-3.249, -3.7891) end of major axis (-3.2942, -3.8786) minor radius 0.0986 (-3.3378, -3.8343) -> (-3.3465, -3.8069) cw
  spline S201 degree 2 poles (-3.3378, -3.8343) (-3.2562, -4.003) (-3.1644, -4.0883) knots 0 0 0 1 1 1
  spline S202 degree 2 poles (-3.1644, -4.0883) (-3.097, -4.1509) (-3.0128, -4.2269) knots 0 0 0 1 1 1
  spline S203 degree 2 poles (-3.0128, -4.2269) (-2.9673, -4.2679) (-2.9153, -4.2969) knots 0 0 0 1 1 1
  spline S204 degree 2 poles (-2.9153, -4.2969) (-2.8253, -4.347) (-2.7552, -4.4201) knots 0 0 0 1 1 1
  ellipse E73 centre (-2.6593, -4.329) end of major axis (-2.7893, -4.355) minor radius 0.1313 (-2.7074, -4.4516) -> (-2.7552, -4.4201) cw
  spline S205 degree 2 poles (-2.7074, -4.4516) (-2.638, -4.478) (-2.5579, -4.5341) knots 0 0 0 1 1 1
  spline S206 degree 3 poles (-2.5579, -4.5341) (-2.5012, -4.5736) (-2.4501, -4.5935) (-2.3918, -4.6055) knots 0 0 0 0 1 1 1 1
  spline S207 degree 2 poles (-2.3918, -4.6055) (-2.2724, -4.6301) (-2.1771, -4.6185) knots 0 0 0 1 1 1
  spline S208 degree 3 poles (-2.1771, -4.6185) (-2.1067, -4.61) (-2.0542, -4.6242) (-1.983, -4.6131) knots 0 0 0 0 1 1 1 1
  ellipse E74 centre (-1.9617, -4.7283) end of major axis (-2.0428, -4.6426) minor radius 0.1152 (-1.983, -4.6131) -> (-1.9368, -4.6149) cw
  spline S209 degree 2 poles (-1.9368, -4.6149) (-1.8356, -4.6393) (-1.7527, -4.6682) knots 0 0 0 1 1 1
  spline S210 degree 2 poles (-1.7527, -4.6682) (-1.6664, -4.6985) (-1.6077, -4.6995) knots 0 0 0 1 1 1
  spline S211 degree 2 poles (-1.6077, -4.6995) (-1.5089, -4.7013) (-1.457, -4.7039) knots 0 0 0 1 1 1
  ellipse E75 centre (-1.4417, -4.5075) end of major axis (-1.5763, -4.6549) minor radius 0.1929 (-1.4157, -4.7014) -> (-1.457, -4.7039) cw
  spline S212 degree 2 poles (-1.4157, -4.7014) (-1.2135, -4.666) (-0.8215, -4.5958) knots 0 0 0 1 1 1
  spline S213 degree 3 poles (-0.8215, -4.5958) (-0.7493, -4.5829) (-0.6698, -4.5863) (-0.6101, -4.6097) knots 0 0 0 0 1 1 1 1
  spline S214 degree 2 poles (-0.6101, -4.6097) (-0.4863, -4.6584) (-0.4774, -4.6609) knots 0 0 0 1 1 1
  spline S215 degree 2 poles (-0.4774, -4.6609) (-0.3743, -4.689) (-0.246, -4.6589) knots 0 0 0 1 1 1
  ellipse E76 centre (-0.24, -4.6668) end of major axis (-0.2497, -4.6618) minor radius 0.0074 (-0.246, -4.6589) -> (-0.2429, -4.6585) cw
  spline S216 degree 2 poles (-0.5296, -3.3526) (-0.4633, -3.3285) (-0.4684, -3.2645) knots 0 0 0 1 1 1
  spline S217 degree 3 poles (-0.4684, -3.2645) (-0.4741, -3.194) (-0.4749, -3.1535) (-0.4893, -3.094) knots 0 0 0 0 1 1 1 1
  spline S218 degree 2 poles (-0.4893, -3.094) (-0.5182, -2.9755) (-0.5245, -2.9398) knots 0 0 0 1 1 1
  spline S219 degree 2 poles (-0.5245, -2.9398) (-0.7697, -1.5399) (-0.8394, -1.1539) knots 0 0 0 1 1 1
  spline S220 degree 2 poles (-0.8394, -1.1539) (-0.857, -1.0558) (-0.8513, -0.9718) knots 0 0 0 1 1 1
  spline S221 degree 2 poles (-0.8513, -0.9718) (-0.849, -0.9375) (-0.8547, -0.9035) knots 0 0 0 1 1 1
  spline S222 degree 2 poles (-0.8547, -0.9035) (-0.921, -0.5172) (-1.0323, 0.1078) knots 0 0 0 1 1 1
  spline S223 degree 2 poles (-1.0323, 0.1078) (-1.0371, 0.135) (-1.0273, 0.2197) knots 0 0 0 1 1 1
  ellipse E77 centre (-1.056, 0.2181) end of major axis (-1.0762, 0.1937) minor radius 0.0268 (-1.0274, 0.2265) -> (-1.0273, 0.2197) cw
  line L22 (-1.0274, 0.2265) -> (-1.048, 0.3684)
  ellipse E78 centre (-0.9174, 0.3843) end of major axis (-1.0125, 0.4783) minor radius 0.1302 (-1.048, 0.3684) -> (-1.0486, 0.4024) cw
  line L23 (-1.0486, 0.4024) -> (-1.0422, 0.4622)
  ellipse E79 centre (-1.0994, 0.4697) end of major axis (-1.1404, 0.5106) minor radius 0.0573 (-1.0423, 0.4765) -> (-1.0422, 0.4622) cw
  line L24 (-1.0423, 0.4765) -> (-1.0563, 0.5837)
  ellipse E80 centre (-1.029, 0.5906) end of major axis (-1.0479, 0.5675) minor radius 0.0257 (-1.0563, 0.5837) -> (-1.0564, 0.588) cw
  spline S224 degree 2 poles (-1.0564, 0.588) (-1.0462, 0.667) (-1.0521, 0.709) knots 0 0 0 1 1 1
  spline S225 degree 2 poles (-1.0521, 0.709) (-1.0579, 0.7499) (-1.0509, 0.8026) knots 0 0 0 1 1 1
  spline S226 degree 2 poles (-1.0509, 0.8026) (-1.0461, 0.8386) (-1.0546, 0.9012) knots 0 0 0 1 1 1
  ellipse E81 centre (-0.9093, 0.9167) end of major axis (-1.0134, 1.0227) minor radius 0.1446 (-1.0546, 0.9012) -> (-1.0547, 0.939) cw
  line L25 (-1.0547, 0.939) -> (-1.0473, 0.996)
  ellipse E82 centre (-1.0774, 0.9995) end of major axis (-1.0987, 0.9779) minor radius 0.0302 (-1.0474, 1.0037) -> (-1.0473, 0.996) cw
  line L26 (-1.0474, 1.0037) -> (-1.066, 1.1297)
  ellipse E83 centre (-0.9739, 1.1469) end of major axis (-1.0392, 1.0781) minor radius 0.0915 (-1.066, 1.1297) -> (-1.0662, 1.1559) cw
  line L27 (-1.0662, 1.1559) -> (-1.0575, 1.2195)
  ellipse E84 centre (-1.0722, 1.2194) end of major axis (-1.0826, 1.2069) minor radius 0.0138 (-1.0576, 1.2244) -> (-1.0575, 1.2195) cw
  spline S227 degree 2 poles (-1.0576, 1.2244) (-1.0739, 1.3336) (-1.0916, 1.4338) knots 0 0 0 1 1 1
  spline S228 degree 2 poles (-1.0916, 1.4338) (-1.3915, 3.1365) (-1.4638, 3.544) knots 0 0 0 1 1 1
  spline S229 degree 3 poles (-1.4638, 3.544) (-1.4808, 3.6405) (-1.622, 3.7414) (-1.7089, 3.7877) knots 0 0 0 0 1 1 1 1
  ellipse E85 centre (-1.7512, 3.7128) end of major axis (-1.8272, 3.6711) minor radius 0.0844 (-1.7444, 3.7976) -> (-1.7089, 3.7877) cw
  spline S230 degree 2 poles (-1.7444, 3.7976) (-1.9026, 3.8057) (-1.9686, 3.7926) knots 0 0 0 1 1 1
  spline S231 degree 2 poles (-1.9686, 3.7926) (-2.1162, 3.7636) (-2.4019, 3.7157) knots 0 0 0 1 1 1
  ellipse E86 centre (-2.4132, 3.7581) end of major axis (-2.4491, 3.7869) minor radius 0.0404 (-2.4019, 3.7157) -> (-2.4094, 3.7154) cw
  line L28 (-2.4094, 3.7154) -> (-2.5735, 3.7219)
  ellipse E87 centre (-2.5733, 3.7217) end of major axis (-2.5741, 3.722) minor radius 0.0002 (-2.5735, 3.7219) -> (-2.5735, 3.7219) cw
  spline S232 degree 2 poles (-2.5733, 3.7217) (-2.6316, 3.7389) (-2.677, 3.7634) knots 0 0 0 1 1 1
  spline S233 degree 3 poles (-2.677, 3.7634) (-2.7314, 3.7926) (-2.8022, 3.8216) (-2.8598, 3.7898) knots 0 0 0 0 1 1 1 1
  spline S234 degree 3 poles (-2.8598, 3.7898) (-2.9455, 3.7426) (-2.9868, 3.666) (-2.9878, 3.5702) knots 0 0 0 0 1 1 1 1
  spline S235 degree 2 poles (-2.9878, 3.5702) (-2.9882, 3.5347) (-2.9931, 3.4876) knots 0 0 0 1 1 1
  ellipse E88 centre (-2.841, 3.4756) end of major axis (-2.9463, 3.3615) minor radius 0.151 (-2.9921, 3.4473) -> (-2.9931, 3.4876) cw
  spline S236 degree 2 poles (-2.9921, 3.4473) (-2.9846, 3.4004) (-2.9679, 3.2984) knots 0 0 0 1 1 1
  spline S237 degree 2 poles (-2.9679, 3.2984) (-2.9617, 3.2596) (-2.9295, 3.1691) knots 0 0 0 1 1 1
  spline S238 degree 2 poles (-2.9295, 3.1691) (-2.9046, 3.0995) (-2.889, 3.0116) knots 0 0 0 1 1 1
  spline S239 degree 2 poles (-2.889, 3.0116) (-2.5703, 1.2228) (-2.4842, 0.7075) knots 0 0 0 1 1 1
  spline S240 degree 2 poles (-2.4842, 0.7075) (-2.4657, 0.5973) (-2.4526, 0.4519) knots 0 0 0 1 1 1
  spline S241 degree 2 poles (-2.4526, 0.4519) (-2.4389, 0.2989) (-2.4208, 0.1968) knots 0 0 0 1 1 1
  spline S242 degree 2 poles (-2.4208, 0.1968) (-2.2831, -0.5856) (-2.2824, -0.5893) knots 0 0 0 1 1 1
  spline S243 degree 2 poles (-2.2824, -0.5893) (-2.2707, -0.6491) (-2.2766, -0.6913) knots 0 0 0 1 1 1
  spline S244 degree 3 poles (-2.2766, -0.6913) (-2.2836, -0.7413) (-2.2784, -0.7637) (-2.2709, -0.8228) knots 0 0 0 0 1 1 1 1
  ellipse E89 centre (-2.409, -0.8459) end of major axis (-2.5095, -0.9461) minor radius 0.1364 (-2.2709, -0.8228) -> (-2.2718, -0.8641) cw
  spline S245 degree 2 poles (-2.2718, -0.8641) (-2.2823, -0.9252) (-2.2684, -0.9976) knots 0 0 0 1 1 1